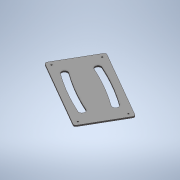
# Autodesk Inventor part: Tempat Batere
Saved by Autodesk Inventor 2020 (Build 240168000, 168)
## iProperties
Created: 2020-03-27
Part Number: Tempat Batere
Material: Generic
Document SubType Name: Modeling
Designer: Muhyidin
Density: 1 g/cm^3
Appearance: Carbon Fiber
Author: Muhyidin
Autodesk Inventor part; units mm, degrees
ref_plane "YZ Plane" through (0, 0, 0) normal (1, 0, 0) x (0, 1, 0)
ref_plane "XZ Plane" through (0, 0, 0) normal (0, 1, 0) x (-1, 0, 0)
ref_plane "XY Plane" through (0, 0, 0) normal (0, 0, 1) x (1, 0, 0)
sketch "Sketch1" plane through (0, 0, 0) normal (0, 1, 0) x (-1, 0, 0)
  circle A0 centre (98.9102, -4.6824) radius 1.6
  circle A1 centre (53.5102, -83.3176) radius 1.6
  circle A2 centre (-98.9102, 4.6824) radius 1.6
  circle A3 centre (-53.5102, 83.3176) radius 1.6
  line L0 (107.5705, -9.6824) -> (62.1705, -88.3176)
  line L1 (-62.1705, 88.3176) -> (-107.5705, 9.6824)
  line L2 (107.5705, -9.6824) -> (112.5705, -1.0222)
  line L3 (112.5705, -1.0222) -> (-57.1705, 96.9778)
  line L4 (112.5705, -1.0222) -> (308.5705, -1.0222) construction
  line L5 (-57.1705, 96.9778) -> (-62.1705, 88.3176)
  line L6 (62.1705, -88.3176) -> (57.1705, -96.9778)
  line L7 (57.1705, -96.9778) -> (-112.5705, 1.0222)
  line L8 (-112.5705, 1.0222) -> (-107.5705, 9.6824)
  line L9 (-15, -25.9808) -> (43, -25.9808) construction
  arc A4 (69.6208, 3.0607) -> (-32.1598, 61.8238) centre (-268.5566, -465.1538) ccw
  arc A5 (60.8381, -9.0992) -> (-38.2992, 48.1377) centre (-268.5566, -465.1538) ccw
  arc A6 (60.8381, -9.0992) -> (69.6208, 3.0607) centre (65.2295, -3.0192) ccw
  arc A7 (-32.1598, 61.8238) -> (-38.2992, 48.1377) centre (-35.2295, 54.9808) ccw
  arc A8 (69.6208, 3.0607) -> (-32.1598, 61.8238) centre (-268.5566, -465.1538) ccw
  arc A9 (60.8381, -9.0992) -> (-38.2992, 48.1377) centre (-268.5566, -465.1538) ccw
  arc A10 (-32.1598, 61.8238) -> (-38.2992, 48.1377) centre (-35.2295, 54.9808) ccw
  arc A11 (60.8381, -9.0992) -> (69.6208, 3.0607) centre (65.2295, -3.0192) ccw
  arc A12 (-69.6208, -3.0607) -> (32.1598, -61.8238) centre (268.5566, 465.1538) ccw
  arc A13 (-60.8381, 9.0992) -> (38.2992, -48.1377) centre (268.5566, 465.1538) ccw
  arc A14 (-60.8381, 9.0992) -> (-69.6208, -3.0607) centre (-65.2295, 3.0192) ccw
  arc A15 (32.1598, -61.8238) -> (38.2992, -48.1377) centre (35.2295, -54.9808) ccw
  point P0 (-50, -7)
  point P1 (-50, -17)
  point P2 (31.0622, -39.8013)
  point P3 (39.7224, -34.8013)
  point P4 (-31.0622, 39.8013)
  point P5 (-39.7224, 34.8013)
  point P6 (50, 7)
  point P7 (50, 17)
  point P8 (18.9378, 46.8013)
  point P9 (10.2776, 51.8013)
  point P10 (-18.9378, -46.8013)
  point P11 (-10.2776, -51.8013)
  point P12 (32.1598, -61.8238)
  dimension "d116" = 10
  dimension "d117" = 10
  dimension "d119" = 150
  dimension "d121" = 90
  dimension "d134" = 15
  constraints: 24 point on circle, 20 end point, 16 centre point, 4 tangent, 2 horizontal, 1 collinear, 1 equal length, 1 perpendicular
  measures "d116" distance of A0.centre L0.start
  measures "d117" distance of A3.centre L1.start
  measures "d119" angle of L4 L3
  measures "d121" angle of L6 L7
  measures "d134" diameter of A7
extrude "Extrusion5" add sketch "Sketch1" along normal blind 3
fillet "Fillet4" radius 5 4 edges at (57.1705, 1.5, 96.9778) (112.5705, 1.5, 1.0222) (-112.5705, 1.5, -1.0222) (-57.1705, 1.5, -96.9778)
body "Solid5"
